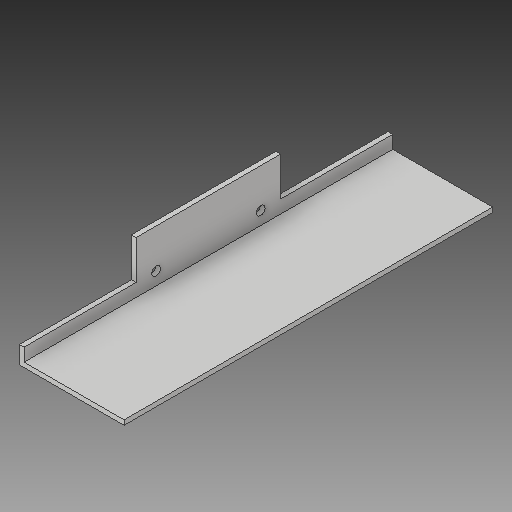
# Autodesk Inventor part: fitplate
Saved by Autodesk Inventor 2018 (Build 220112000, 112)
## iProperties
Created: 2017-04-13
Part Number: fitplate
Material: Generic
Document SubType Name: Modeling
Designer: steve
Density: 1 g/cm^3
Appearance: Default
Mass: 8.99226 g
Surface Area: 118.404 cm^2
Volume: 8.99226 cm^3
Vendor: Rhoban
Author: steve
Autodesk Inventor part; units mm, degrees
ref_plane "YZ Plane" through (0, 0, 0) normal (1, 0, 0) x (0, 1, 0)
ref_plane "XZ Plane" through (0, 0, 0) normal (0, 1, 0) x (-1, 0, 0)
ref_plane "XY Plane" through (0, 0, 0) normal (0, 0, 1) x (1, 0, 0)
sketch "Sketch1" plane through (0, 0, 0) normal (0, 1, 0) x (-1, 0, 0)
  line L0 (-17.75, 62.5) -> (17.75, 62.5)
  line L1 (17.75, 62.5) -> (17.75, -62.5)
  line L2 (17.75, -62.5) -> (-17.75, -62.5)
  line L3 (-17.75, -62.5) -> (-17.75, 62.5)
  line L4 (-17.75, 62.5) -> (17.75, -62.5) construction
  line L5 (17.75, 62.5) -> (-17.75, -62.5) construction
  point P0 (0, 0)
  dimension "d0" = 35.5
  dimension "d1" = 125
  constraints: 12 end point, 2 midpoint, 2 parallel, 1 horizontal, 1 perpendicular
  measures "d0" distance of L1.end L2.end
  measures "d1" distance of L0.end L1.end
extrude "Extrusion1" add sketch "Sketch1" along normal blind 1.6
sketch "Sketch2" plane through (0, 1.6, 0) normal (0, 1, 0) x (1, 0, 0)
  line L0 (17.75, 62.5) -> (-17.75, 62.5) projected
  line L1 (-17.75, -62.5) -> (17.75, -62.5) projected
  line L2 (-17.75, 62.5) -> (-16.15, 62.5)
  line L3 (-16.15, 62.5) -> (-16.15, -62.5)
  line L4 (-16.15, -62.5) -> (-17.75, -62.5)
  line L5 (-17.75, -62.5) -> (-17.75, 62.5)
  point P0 (0, 0)
  dimension "d4" = 1.6
  constraints: 8 end point, 2 parallel, 1 horizontal, 1 perpendicular, 1 point on line
  measures "d4" distance between parallel lines of L5 L3
extrude "Extrusion2" add sketch "Sketch2" along normal blind 17.6
sketch "Sketch3" plane through (-17.75, 0, -62.5) normal (-1, 0, 0) x (0, 0, 1)
  line L0 (62.5, 0) -> (62.5, 72.1121) construction
  line L1 (98.5, 0) -> (26.5, 0) construction
  line L2 (26.5, 0) -> (26.5, 19.2) construction
  line L3 (26.5, 19.2) -> (98.5, 19.2) construction
  line L4 (98.5, 19.2) -> (98.5, 0) construction
  line L5 (98.5, 0) -> (26.5, 19.2) construction
  line L6 (26.5, 0) -> (98.5, 19.2) construction
  line L7 (0, 19.2) -> (125, 19.2) construction
  line L8 (125, 0) -> (0, 0) construction
  line L9 (125, 19.2) -> (87, 19.2)
  line L10 (87, 19.2) -> (87, 6)
  line L11 (87, 6) -> (125, 6)
  line L12 (125, 6) -> (125, 19.2)
  line L13 (0, 19.2) -> (38, 19.2)
  line L14 (38, 19.2) -> (38, 6)
  line L15 (38, 6) -> (0, 6)
  line L16 (0, 6) -> (0, 19.2)
  point P0 (62.5, 9.6)
  dimension "d7" = 72
  dimension "d8" = 38
  dimension "d9" = 6
  constraints: 30 end point, 4 parallel, 3 symmetric about line, 2 collinear, 2 horizontal, 2 midpoint, 2 perpendicular, 1 point on line, 1 vertical
  measures "d7" distance between parallel lines of L4 L2
  measures "d8" distance between parallel lines of L12 L10
  measures "d9" distance between parallel lines of L8 L11
extrude "Extrusion3" cut sketch "Sketch3" against normal through all
sketch "Sketch4" plane through (-17.75, 0, -62.5) normal (-1, 0, 0) x (0, 0, 1)
  line L0 (62.5, 0) -> (62.5, 59.5527) construction
  line L1 (44.75, 6) -> (80.25, 6) construction
  line L2 (80.25, 6) -> (80.25, 0) construction
  line L3 (80.25, 0) -> (44.75, 0) construction
  line L4 (44.75, 0) -> (44.75, 6) construction
  line L5 (44.75, 6) -> (80.25, 0) construction
  line L6 (80.25, 6) -> (44.75, 0) construction
  line L7 (125, 0) -> (0, 0) construction
  point P0 (62.5, 3)
  dimension "d12" = 6
  dimension "d13" = 35.5
  constraints: 14 end point, 2 coincident, 2 midpoint, 2 parallel, 1 collinear, 1 horizontal, 1 perpendicular, 1 point on line, 1 vertical
  measures "d12" distance of L1.end L2.end
  measures "d13" distance of L1.start L1.end
hole "Hole1" at (-17.75, 6, 17.75) at (-17.75, 6, -17.75) direction (1, 0, 0) diameter 3 end through all
body "Solid1"
